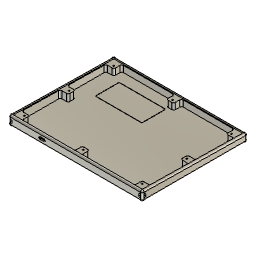
case (Autodesk Fusion 360 design; units mm, degrees)
Autodesk Fusion 360 part; units mm, degrees
sketch "Sketch1" plane through (0, 0, 0) normal (0, 0, 1) x (1, 0, 0)
  line L0 (0, 0) -> (294.692, 0)
  line L1 (294.692, 0) -> (294.692, 230.4)
  line L2 (294.692, 230.4) -> (0, 230.4)
  line L3 (0, 230.4) -> (0, 0)
  line L4 (-4, 234.4) -> (298.692, 234.4)
  line L5 (298.692, 234.4) -> (298.692, -4)
  line L6 (298.692, -4) -> (-4, -4)
  line L7 (-4, -4) -> (-4, 234.4)
  line L8 (4, 226.4) -> (290.692, 226.4)
  line L9 (290.692, 226.4) -> (290.692, 4)
  line L10 (290.692, 4) -> (4, 4)
  line L11 (4, 4) -> (4, 226.4)
  line L12 (4, 226.4) -> (20, 226.4)
  line L13 (20, 226.4) -> (20, 210.4)
  line L14 (20, 210.4) -> (4, 210.4)
  line L15 (4, 210.4) -> (4, 226.4)
  line L16 (4, 4) -> (20, 4)
  line L17 (20, 4) -> (20, 20)
  line L18 (20, 20) -> (4, 20)
  line L19 (4, 20) -> (4, 4)
  line L20 (290.692, 4) -> (274.692, 4)
  line L21 (274.692, 4) -> (274.692, 20)
  line L22 (274.692, 20) -> (290.692, 20)
  line L23 (290.692, 20) -> (290.692, 4)
  line L24 (290.692, 226.4) -> (274.692, 226.4)
  line L25 (274.692, 226.4) -> (274.692, 210.4)
  line L26 (274.692, 210.4) -> (290.692, 210.4)
  line L27 (290.692, 210.4) -> (290.692, 226.4)
  line L28 (4, 226.4) -> (290.692, 4) construction
  line L29 (4, 4) -> (290.692, 226.4) construction
  line L30 (147.346, 226.4) -> (147.346, 4) construction
  line L31 (4, 115.2) -> (290.692, 115.2) construction
  line L32 (4, 123.2) -> (20, 123.2)
  line L33 (20, 123.2) -> (20, 107.2)
  line L34 (20, 107.2) -> (4, 107.2)
  line L35 (4, 107.2) -> (4, 123.2)
  line L36 (139.346, 226.4) -> (155.346, 226.4)
  line L37 (155.346, 226.4) -> (155.346, 210.4)
  line L38 (155.346, 210.4) -> (139.346, 210.4)
  line L39 (139.346, 210.4) -> (139.346, 226.4)
  line L40 (290.692, 123.2) -> (274.692, 123.2)
  line L41 (274.692, 123.2) -> (274.692, 107.2)
  line L42 (274.692, 107.2) -> (290.692, 107.2)
  line L43 (290.692, 107.2) -> (290.692, 123.2)
  line L44 (139.346, 4) -> (155.346, 4)
  line L45 (155.346, 4) -> (155.346, 20)
  line L46 (155.346, 20) -> (139.346, 20)
  line L47 (139.346, 20) -> (139.346, 4)
  line L48 (2, 228.4) -> (292.692, 228.4)
  line L49 (292.692, 228.4) -> (292.692, 2)
  line L50 (292.692, 2) -> (2, 2)
  line L51 (2, 2) -> (2, 228.4)
  line L52 (20, 210.4) -> (2, 210.4)
  line L53 (2, 210.4) -> (2, 228.4)
  line L54 (2, 228.4) -> (20, 228.4)
  line L55 (20, 228.4) -> (20, 210.4)
  line L56 (20, 20) -> (2, 20)
  line L57 (2, 20) -> (2, 2)
  line L58 (2, 2) -> (20, 2)
  line L59 (20, 2) -> (20, 20)
  line L60 (274.692, 20) -> (292.692, 20)
  line L61 (292.692, 20) -> (292.692, 2)
  line L62 (292.692, 2) -> (274.692, 2)
  line L63 (274.692, 2) -> (274.692, 20)
  line L64 (274.692, 210.4) -> (292.692, 210.4)
  line L65 (292.692, 210.4) -> (292.692, 228.4)
  line L66 (292.692, 228.4) -> (274.692, 228.4)
  line L67 (274.692, 228.4) -> (274.692, 210.4)
  line L68 (139.346, 210.4) -> (155.346, 210.4)
  line L69 (155.346, 210.4) -> (155.346, 228.4)
  line L70 (155.346, 228.4) -> (139.346, 228.4)
  line L71 (139.346, 228.4) -> (139.346, 210.4)
  line L72 (274.692, 107.2) -> (292.692, 107.2)
  line L73 (292.692, 107.2) -> (292.692, 123.2)
  line L74 (292.692, 123.2) -> (274.692, 123.2)
  line L75 (274.692, 123.2) -> (274.692, 107.2)
  line L76 (155.346, 20) -> (139.346, 20)
  line L77 (139.346, 20) -> (139.346, 2)
  line L78 (139.346, 2) -> (155.346, 2)
  line L79 (155.346, 2) -> (155.346, 20)
  line L80 (20, 107.2) -> (2, 107.2)
  line L81 (2, 107.2) -> (2, 123.2)
  line L82 (2, 123.2) -> (20, 123.2)
  line L83 (20, 123.2) -> (20, 107.2)
  line L84 (0, 230.4) -> (37.901, 230.4) construction
  line L85 (37.901, 230.4) -> (37.901, 204.499) construction
  line L86 (37.901, 204.499) -> (0, 204.499) construction
  line L87 (0, 204.499) -> (0, 230.4) construction
  line L88 (37.901, 204.499) -> (143.109, 204.499)
  line L89 (143.109, 204.499) -> (143.109, 150.891)
  line L90 (143.109, 150.891) -> (37.901, 150.891)
  line L91 (37.901, 150.891) -> (37.901, 204.499)
  dimension "d1" = 294.692
  dimension "d2" = 230.4
  dimension "d3" = 4
  dimension "d4" = 4
  dimension "d5" = 4
  dimension "d6" = 4
  dimension "d7" = 4
  dimension "d8" = 4
  dimension "d9" = 4
  dimension "d10" = 4
  dimension "d11" = 16
  dimension "d12" = 16
  dimension "d13" = 16
  dimension "d14" = 16
  dimension "d15" = 16
  dimension "d16" = 16
  dimension "d17" = 16
  dimension "d18" = 16
  dimension "d19" = 16
  dimension "d20" = 16
  dimension "d21" = 16
  dimension "d22" = 16
  dimension "d23" = 16
  dimension "d24" = 16
  dimension "d25" = 16
  dimension "d26" = 16
  dimension "d27" = 2
  dimension "d28" = 2
  dimension "d29" = 2
  dimension "d30" = 2
  dimension "d33" = 16
  dimension "d34" = 16
  dimension "d35" = 16
  dimension "d36" = 16
  dimension "d150" = 37.901
  dimension "d151" = 25.901
  dimension "d152" = 105.208
  dimension "d153" = 53.608
  constraint horizontal L0
  constraint vertical L1
  constraint horizontal L2
  constraint vertical L3
  constraint coincident L0.start L3.end
  constraint horizontal L4
  constraint vertical L5
  constraint horizontal L6
  constraint vertical L7
  constraint horizontal L8
  constraint vertical L9
  constraint horizontal L10
  constraint vertical L11
  constraint horizontal L12
  constraint vertical L13
  constraint horizontal L14
  constraint vertical L15
  constraint horizontal L16
  constraint vertical L17
  constraint horizontal L18
  constraint vertical L19
  constraint horizontal L20
  constraint vertical L21
  constraint horizontal L22
  constraint vertical L23
  constraint horizontal L24
  constraint vertical L25
  constraint horizontal L26
  constraint vertical L27
  constraint midpoint L8 L30.start
  constraint midpoint L10 L30.end
  constraint midpoint L11 L31.start
  constraint midpoint L9 L31.end
  constraint horizontal L32
  constraint vertical L33
  constraint horizontal L34
  constraint vertical L35
  constraint coincident L11 L32.start
  constraint symmetric L31 L32 L34
  constraint horizontal L36
  constraint vertical L37
  constraint horizontal L38
  constraint vertical L39
  constraint coincident L8 L36.start
  constraint symmetric L30 L37 L39
  constraint horizontal L40
  constraint vertical L41
  constraint horizontal L42
  constraint vertical L43
  constraint coincident L9 L40.start
  constraint symmetric L31 L40 L42
  constraint horizontal L44
  constraint vertical L45
  constraint horizontal L46
  constraint vertical L47
  constraint coincident L10 L44.start
  constraint symmetric L30 L45 L47
  constraint horizontal L48
  constraint vertical L49
  constraint horizontal L50
  constraint vertical L51
  constraint horizontal L52
  constraint vertical L53
  constraint horizontal L54
  constraint vertical L55
  constraint horizontal L56
  constraint vertical L57
  constraint horizontal L58
  constraint vertical L59
  constraint horizontal L60
  constraint vertical L61
  constraint horizontal L62
  constraint vertical L63
  constraint horizontal L64
  constraint vertical L65
  constraint horizontal L66
  constraint vertical L67
  constraint horizontal L68
  constraint vertical L69
  constraint horizontal L70
  constraint vertical L71
  constraint horizontal L72
  constraint vertical L73
  constraint horizontal L74
  constraint vertical L75
  constraint coincident L49 L73.end
  constraint horizontal L76
  constraint vertical L77
  constraint horizontal L78
  constraint vertical L79
  constraint horizontal L80
  constraint vertical L81
  constraint horizontal L82
  constraint vertical L83
  constraint horizontal L84
  constraint vertical L85
  constraint horizontal L86
  constraint vertical L87
  constraint horizontal L88
  constraint vertical L89
  constraint horizontal L90
  constraint vertical L91
  measures "d1" distance of L0.start L0.end
  measures "d2" distance of L0.start L2.end
  measures "d3" distance of L3 L7
  measures "d4" distance of L2 L4
  measures "d5" distance of L0 L6
  measures "d6" distance of L1 L5
  measures "d7" distance of L3 L11
  measures "d8" distance of L2 L8
  measures "d9" distance of L1 L9
  measures "d10" distance of L0 L10
  measures "d11" distance of L8.start L12.end
  measures "d12" distance of L8.start L14.end
  measures "d13" distance of L10.end L16.end
  measures "d14" distance of L10.end L18.end
  measures "d15" distance of L9.end L20.end
  measures "d16" distance of L9.end L22.end
  measures "d17" distance of L8.end L24.end
  measures "d18" distance of L8.end L26.end
  measures "d19" distance of L32.start L32.end
  measures "d20" distance of L32.start L34.end
  measures "d21" distance of L36.start L36.end
  measures "d22" distance of L36.start L38.end
  measures "d23" distance of L40.start L40.end
  measures "d24" distance of L40.start L42.end
  measures "d25" distance of L44.start L44.end
  measures "d26" distance of L44.start L46.end
  measures "d27" distance of L3 L51
  measures "d28" distance of L2 L48
  measures "d29" distance of L0 L50
  measures "d30" distance of L1 L49
  measures "d33" distance of L38.end L37.end
  measures "d34" distance of L41.end L40.end
  measures "d35" distance of L45.end L46.end
  measures "d36" distance of L33.end L32.end
  measures "d150" distance of L2.end L84.end
  measures "d151" distance of L2.end L86.end
  measures "d152" distance of L85.end L88.end
  measures "d153" distance of L85.end L90.end
extrude "Extrude1" add sketch "Sketch1" against normal blind 1.5 contours L0 L1 L2 L3 | L4 L5 L6 L7 | L8 L11 L12 L15 L48 L51 L52 L53 L54 L55 | L8 L11 L12 L13 L14 L15 L52 L55 | L8 L48 L55 L71 | L8 L9 L10 L11 L13 L14 L17 L18 L21 L22 L25 L26 L32 L33 L34 L37 L38 L39 L40 L41 L42 L45 L46 L47 L52 L55 L56 L59 L60 L63 L64 L67 L68 L69 L71 L72 L74 L75 L76 L77 L79 L80 L82 L83 | L11 L51 L52 L82 | L8 L36 L48 L69 L70 L71 | L8 L36 L37 L38 L39 L68 L69 L71 | L11 L32 L33 L34 L35 L80 L82 L83 | L11 L35 L51 L80 L81 L82 | L8 L48 L67 L69 | L11 L51 L56 L80 | L8 L9 L24 L27 L48 L49 L64 L65 L66 L67 | L8 L9 L24 L25 L26 L27 L64 L67 | L10 L11 L16 L17 L18 L19 L56 L59 | L10 L11 L16 L19 L50 L51 L56 L57 L58 L59 | L9 L49 L64 L74 | L10 L50 L59 L77 | L9 L43 L49 L72 L73 L74 | L9 L40 L41 L42 L43 L72 L74 L75 | L10 L44 L45 L46 L47 L76 L77 L79 | L10 L44 L50 L77 L78 L79 | L9 L49 L60 L72 | L10 L50 L63 L79 | L9 L10 L20 L23 L49 L50 L60 L61 L62 L63 | L9 L10 L20 L21 L22 L23 L60 L63 | L88 L89 L90 L91 makes body 1
extrude "Extrude2" add sketch "Sketch1" along normal blind 18 contours L0 L1 L2 L3 | L4 L5 L6 L7 | L8 L11 L12 L15 L48 L51 L52 L53 L54 L55 | L8 L11 L12 L13 L14 L15 L52 L55 | L8 L36 L48 L69 L70 L71 | L8 L36 L37 L38 L39 L68 L69 L71 | L11 L32 L33 L34 L35 L80 L82 L83 | L11 L35 L51 L80 L81 L82 | L8 L9 L24 L27 L48 L49 L64 L65 L66 L67 | L8 L9 L24 L25 L26 L27 L64 L67 | L10 L11 L16 L17 L18 L19 L56 L59 | L10 L11 L16 L19 L50 L51 L56 L57 L58 L59 | L9 L43 L49 L72 L73 L74 | L9 L40 L41 L42 L43 L72 L74 L75 | L10 L44 L45 L46 L47 L76 L77 L79 | L10 L44 L50 L77 L78 L79 | L9 L10 L20 L23 L49 L50 L60 L61 L62 L63 | L9 L10 L20 L21 L22 L23 L60 L63 bodies 1
sketch "Sketch2" plane through (0, 0, 18) normal (0, 0, 1) x (-1, 0, 0)
  line L0 (-20, -123.2) -> (-2, -123.2)
  line L1 (-2, -123.2) -> (-2, -210.4)
  line L2 (-2, -210.4) -> (-20, -210.4)
  line L3 (-20, -210.4) -> (-20, -228.4)
  line L4 (-20, -228.4) -> (-139.346, -228.4)
  line L5 (-139.346, -228.4) -> (-139.346, -210.4)
  line L6 (-139.346, -210.4) -> (-155.346, -210.4)
  line L7 (-155.346, -210.4) -> (-155.346, -228.4)
  line L8 (-155.346, -228.4) -> (-274.692, -228.4)
  line L9 (-274.692, -228.4) -> (-274.692, -210.4)
  line L10 (-274.692, -210.4) -> (-292.692, -210.4)
  line L11 (-292.692, -210.4) -> (-292.692, -123.2)
  line L12 (-292.692, -123.2) -> (-274.692, -123.2)
  line L13 (-274.692, -123.2) -> (-274.692, -107.2)
  line L14 (-274.692, -107.2) -> (-292.692, -107.2)
  line L15 (-292.692, -107.2) -> (-292.692, -20)
  line L16 (-292.692, -20) -> (-274.692, -20)
  line L17 (-274.692, -20) -> (-274.692, -2)
  line L18 (-274.692, -2) -> (-155.346, -2)
  line L19 (-155.346, -2) -> (-155.346, -20)
  line L20 (-155.346, -20) -> (-139.346, -20)
  line L21 (-139.346, -20) -> (-139.346, -2)
  line L22 (-139.346, -2) -> (-20, -2)
  line L23 (-20, -2) -> (-20, -20)
  line L24 (-20, -20) -> (-2, -20)
  line L25 (-2, -20) -> (-2, -107.2)
  line L26 (-2, -107.2) -> (-20, -107.2)
  line L27 (-20, -107.2) -> (-20, -123.2)
  line L28 (4, 4) -> (-298.692, 4)
  line L29 (-298.692, 4) -> (-298.692, -234.4)
  line L30 (-298.692, -234.4) -> (4, -234.4)
  line L31 (4, -234.4) -> (4, 4)
  line L32 (-294.692, 0) -> (0, 0)
  line L33 (0, 0) -> (0, -230.4)
  line L34 (0, -230.4) -> (-294.692, -230.4)
  line L35 (-294.692, -230.4) -> (-294.692, 0)
  dimension "d39" = 4
  dimension "d40" = 4
  dimension "d41" = 4
  dimension "d42" = 4
  constraint horizontal L32
  constraint vertical L33
  constraint horizontal L34
  constraint vertical L35
  measures "d39" distance of L29 L35
  measures "d40" distance of L28 L32
  measures "d41" distance of L30 L34
  measures "d42" distance of L31 L33
sketch "Sketch3" plane through (298.692, 0, 0) normal (1, 0, 0) x (0, 1, 0)
  line L0 (-4, 18) -> (-4, -1.5)
  line L1 (-4, -1.5) -> (234.4, -1.5)
  line L2 (234.4, -1.5) -> (234.4, 18)
  line L3 (234.4, 18) -> (-4, 18)
  line L4 (234.4, -1.5) -> (234.4, 14)
  line L5 (-4, 18) -> (234.4, 14)
  dimension "d43" = 15.5
  constraint coincident L1.end L2.start
  constraint perpendicular L1 L4
  constraint coincident L0.start L3.end
  measures "d43" distance of L1.end L4.end
extrude "Extrude3" cut sketch "Sketch3" against normal through all contours L2 L3 L5 bodies 1
extrude "Extrude4" add sketch "Sketch2" along normal blind 3 separate body contours L28 L29 L30 L31 makes body 2
extrude "Extrude5" add 1 faces at (196.4613, 233.0667, 18) along direction (0, 0, -1) through all on bodies 2 bodies 1 2
sketch "Sketch4" plane through (298.692, 0, 0) normal (1, 0, 0) x (0, 1, 0)
  line L0 (234.4, -1.5) -> (234.4, 21)
  line L1 (234.4, 21) -> (-4, 21)
  line L2 (-4, 21) -> (-4, -1.5)
  line L3 (-4, -1.5) -> (234.4, -1.5)
  line L4 (234.4, -1.5) -> (234.4, 17)
  line L5 (234.4, 17) -> (-4, 21)
  dimension "d48" = 18.5
  constraint coincident L0.start L3.end
  constraint perpendicular L3 L4
  constraint coincident L1.end L2.start
  measures "d48" distance of L0.start L4.end
extrude "Extrude6" cut sketch "Sketch4" against normal through all contours L0 L1 L5 bodies 1
sketch "Sketch5" plane through (298.692, 0, 0) normal (1, 0, 0) x (0, 1, 0)
  line L0 (234.4, 17) -> (-4, 21)
  line L1 (-4, 21) -> (-4, -1.5)
  line L2 (-4, -1.5) -> (234.4, -1.5)
  line L3 (234.4, -1.5) -> (234.4, 17)
  line L4 (-4, 9.75) -> (234.4, 9.75) construction
  line L5 (-4, 13.75) -> (0, 13.75)
  line L6 (0, 13.75) -> (0, 5.75)
  line L7 (0, 5.75) -> (-4, 5.75)
  line L8 (-4, 5.75) -> (-4, 13.75)
  line L9 (-4, 13.75) -> (4, 13.75)
  line L10 (4, 13.75) -> (4, 5.75)
  line L11 (4, 5.75) -> (-4, 5.75)
  line L12 (-4, 5.75) -> (-4, 13.75)
  dimension "d50" = 4
  dimension "d51" = 8
  dimension "d52" = 8
  constraint midpoint L1 L4.start
  constraint coincident L3 L4.end
  constraint perpendicular L3 L4
  constraint horizontal L5
  constraint vertical L6
  constraint horizontal L7
  constraint vertical L8
  constraint coincident L1 L5.start
  constraint horizontal L9
  constraint vertical L10
  constraint horizontal L11
  constraint vertical L12
  constraint equal L6 L10
  constraint symmetric L4 L5 L7
  measures "d50" distance of L5.start L5.end
  measures "d51" distance of L5.start L7.end
  measures "d52" distance of L5.start L9.end
sketch "Sketch6" plane through (0, -4, 0) normal (0, -1, 0) x (1, 0, 0)
  line L0 (-4, 21) -> (-4, -1.5)
  line L1 (-4, -1.5) -> (298.692, -1.5)
  line L2 (298.692, -1.5) -> (298.692, 21)
  line L3 (298.692, 21) -> (-4, 21)
  line L4 (298.692, 21) -> (-4, -1.5) construction
  line L5 (-4, 21) -> (298.692, -1.5) construction
  line L6 (147.346, -1.5) -> (147.346, 21) construction
  line L7 (147.346, 21) -> (-4, -1.5) construction
  line L8 (-4, 21) -> (147.346, -1.5) construction
  line L9 (-4, 9.75) -> (147.346, 9.75) construction
  line L10 (-4, 13.75) -> (0, 13.75)
  line L11 (0, 13.75) -> (0, 5.75)
  line L12 (0, 5.75) -> (-4, 5.75)
  line L13 (-4, 5.75) -> (-4, 13.75)
  line L14 (-4, 13.75) -> (4, 13.75)
  line L15 (4, 13.75) -> (4, 5.75)
  line L16 (4, 5.75) -> (-4, 5.75)
  line L17 (-4, 5.75) -> (-4, 13.75)
  line L18 (298.692, 9.75) -> (147.346, 9.75) construction
  line L19 (298.692, 13.75) -> (294.692, 13.75)
  line L20 (294.692, 13.75) -> (294.692, 5.75)
  line L21 (294.692, 5.75) -> (298.692, 5.75)
  line L22 (298.692, 5.75) -> (298.692, 13.75)
  line L23 (298.692, 13.75) -> (290.692, 13.75)
  line L24 (290.692, 13.75) -> (290.692, 5.75)
  line L25 (290.692, 5.75) -> (298.692, 5.75)
  line L26 (298.692, 5.75) -> (298.692, 13.75)
  line L27 (62.173, 12.5) -> (81.173, 12.5)
  line L28 (81.173, 12.5) -> (81.173, 7)
  line L29 (81.173, 7) -> (62.173, 7)
  line L30 (62.173, 7) -> (62.173, 12.5)
  line L31 (71.673, 9.75) -> (71.673, -1.5) construction
  line L32 (66.173, 12.5) -> (77.173, 12.5)
  line L33 (77.173, 12.5) -> (77.173, 7)
  line L34 (77.173, 7) -> (66.173, 7)
  line L35 (66.173, 7) -> (66.173, 12.5)
  circle A0 centre (64.423, 9.7337) radius 1
  circle A1 centre (78.923, 9.7337) radius 1
  dimension "d53" = 4
  dimension "d54" = 8
  dimension "d55" = 8
  dimension "d67" = 4
  dimension "d68" = 8
  dimension "d69" = 8
  dimension "d158" = 19
  dimension "d159" = 5.5
  dimension "d160" = 11
  dimension "d161" = 2
  dimension "d162" = 2
  dimension "d177" = 14.5
  constraint coincident L2.end L3.start
  constraint coincident L0.end L1.start
  constraint coincident L0.start L3.end
  constraint coincident L1.end L2.start
  constraint midpoint L1 L6.start
  constraint midpoint L3 L6.end
  constraint midpoint L0 L9.start
  constraint midpoint L6 L9.end
  constraint horizontal L10
  constraint vertical L11
  constraint horizontal L12
  constraint vertical L13
  constraint coincident L0 L10.start
  constraint horizontal L14
  constraint vertical L15
  constraint horizontal L16
  constraint vertical L17
  constraint equal L11 L15
  constraint symmetric L9 L10 L12
  constraint midpoint L2 L18.start
  constraint horizontal L19
  constraint vertical L20
  constraint horizontal L21
  constraint vertical L22
  constraint coincident L2 L19.start
  constraint horizontal L23
  constraint vertical L24
  constraint horizontal L25
  constraint vertical L26
  constraint equal L20 L24
  constraint symmetric L18 L19 L21
  constraint horizontal L27
  constraint vertical L28
  constraint horizontal L29
  constraint vertical L30
  constraint midpoint L9 L31.start
  constraint coincident L1 L31.end
  constraint perpendicular L1 L31
  constraint symmetric L28 L30 L31
  constraint symmetric L9 L27 L29
  constraint horizontal L32
  constraint vertical L33
  constraint horizontal L34
  constraint vertical L35
  constraint coincident L27 L32.start
  constraint equal L30 L35
  constraint symmetric L31 L33 L35
  constraint symmetric L31 A0.centre A1.centre
  measures "d53" distance of L10.start L10.end
  measures "d54" distance of L10.start L12.end
  measures "d55" distance of L10.start L14.end
  measures "d67" distance of L19.start L19.end
  measures "d68" distance of L19.start L21.end
  measures "d69" distance of L19.start L23.end
  measures "d158" distance of L27.start L27.end
  measures "d159" distance of L27.start L29.end
  measures "d160" distance of L32.start L32.end
  measures "d161" diameter of A0
  measures "d162" diameter of A1
  measures "d177" distance of A0.centre A1.centre
sketch "Sketch7" plane through (-4, 0, 0) normal (-1, 0, 0) x (0, -1, 0)
  line L0 (4, 21) -> (-234.4, 17)
  line L1 (-234.4, 17) -> (-234.4, -1.5)
  line L2 (-234.4, -1.5) -> (4, -1.5)
  line L3 (4, -1.5) -> (4, 21)
  line L4 (4, 9.75) -> (-234.4, 9.75) construction
  line L5 (4, 13.75) -> (0, 13.75)
  line L6 (0, 13.75) -> (0, 5.75)
  line L7 (0, 5.75) -> (4, 5.75)
  line L8 (4, 5.75) -> (4, 13.75)
  line L9 (4, 13.75) -> (-4, 13.75)
  line L10 (-4, 13.75) -> (-4, 5.75)
  line L11 (-4, 5.75) -> (4, 5.75)
  line L12 (4, 5.75) -> (4, 13.75)
  dimension "d58" = 4
  dimension "d59" = 8
  dimension "d60" = 8
  constraint midpoint L3 L4.start
  constraint coincident L1 L4.end
  constraint perpendicular L1 L4
  constraint horizontal L5
  constraint vertical L6
  constraint horizontal L7
  constraint vertical L8
  constraint coincident L3 L5.start
  constraint horizontal L9
  constraint vertical L10
  constraint horizontal L11
  constraint vertical L12
  constraint equal L6 L10
  constraint symmetric L4 L5 L7
  measures "d58" distance of L5.start L5.end
  measures "d59" distance of L5.start L7.end
  measures "d60" distance of L5.start L9.end
fillet "Fillet1" radius 4 28 edges at (20, 228.4, 7.0503) (20, 210.4, 7.2013) (2, 210.4, 7.2013) (20, 123.2, 7.9329) (2, 123.2, 7.9329) (2, 107.2, 8.0671) (20, 107.2, 8.0671) (2, 20, 8.7987) (20, 20, 8.7987) (20, 2, 8.9497) (139.346, 20, 8.7987) (139.346, 2, 8.9497) (155.346, 20, 8.7987) (155.346, 2, 8.9497) (274.692, 20, 8.7987) (274.692, 2, 8.9497) (292.692, 20, 8.7987) (292.692, 107.2, 8.0671) (274.692, 107.2, 8.0671) (274.692, 123.2, 7.9329) (292.692, 123.2, 7.9329) (292.692, 210.4, 7.2013) (274.692, 210.4, 7.2013) (274.692, 228.4, 7.0503) (155.346, 228.4, 7.0503) (139.346, 228.4, 7.0503) (139.346, 210.4, 7.2013) (155.346, 210.4, 7.2013) on bodies 1
fillet "Fillet2" radius 2 4 edges at (294.692, 230.4, 15.5671) (0, 230.4, 15.5671) (0, 0, 19.4329) (294.692, 0, 19.4329) on bodies 1
fillet "Fillet3" radius 4 4 edges at (-4, -4, 9.75) (298.692, -4, 9.75) (-4, 234.4, 7.75) (298.692, 234.4, 7.75) on bodies 1
extrude "Extrude8" cut sketch "Sketch7" against normal blind 4 contours L6 L9 L10 L11 bodies 1
extrude "Extrude9" cut sketch "Sketch6" against normal blind 8 contours L11 L14 L15 L16 bodies 1
extrude "Extrude10" cut sketch "Sketch5" against normal blind 4 contours L6 L9 L10 L11 bodies 1
extrude "Extrude11" cut sketch "Sketch6" against normal blind 8 contours L20 L23 L24 L25 bodies 1
fillet "Fillet4" radius 2 5 edges at (290.692, 0, 13.75) (294.692, 4, 13.75) (290.692, 0, 5.75) (294.692, 4, 5.75) (290.692, 4, 9.75) on bodies 1
fillet "Fillet5" radius 2 5 edges at (0, 4, 13.75) (4, 0, 13.75) (0, 4, 5.75) (4, 0, 5.75) (4, 4, 9.75) on bodies 1
fillet "Fillet6" radius 4 16 edges at (297.5204, -2.8284, 20.9803) (298.692, 115.2, 19) (297.5204, 233.2284, 17.0197) (147.346, 234.4, 17) (-2.8284, 233.2284, 17.0197) (-4, 115.2, 19) (-2.8284, -2.8284, 20.9803) (147.346, -4, 21) (-2.8284, -2.8284, -1.5) (-4, 115.2, -1.5) (-2.8284, 233.2284, -1.5) (147.346, 234.4, -1.5) (297.5204, 233.2284, -1.5) (298.692, 115.2, -1.5) (297.5204, -2.8284, -1.5) (147.346, -4, -1.5) on bodies 1
hole "Hole1" at (280.692, 14.0008, 17.698) direction (0, -0.016776, -0.999859) diameter 3.332 depth 10 tip angle 118 bodies 1
thread "Thread1" "ISO Metric profile 4.0 M4x0.7 6H" thread offset 0 thread depth 7.4
hole "Hole2" at (147.346, 14.0008, 17.698) direction (0, -0.016776, -0.999859) diameter 3.332 depth 10 tip angle 118 bodies 1
thread "Thread2" "ISO Metric profile 4.0 M4x0.7 6H" thread offset 0 thread depth 7.4
hole "Hole3" at (14, 14.0008, 17.698) direction (0, -0.016776, -0.999859) diameter 3.332 depth 10 tip angle 118 bodies 1
thread "Thread3" "ISO Metric profile 4.0 M4x0.7 6H" thread offset 0 thread depth 7.4
hole "Hole4" at (280.692, 115.1989, 16) direction (0, -0.016776, -0.999859) diameter 3.332 depth 10 tip angle 118 bodies 1
thread "Thread4" "ISO Metric profile 4.0 M4x0.7 6H" thread offset 0 thread depth 7.4
hole "Hole5" at (14, 115.1989, 16) direction (0, -0.016776, -0.999859) diameter 3.332 depth 10 tip angle 118 bodies 1
thread "Thread5" "ISO Metric profile 4.0 M4x0.7 6H" thread offset 0 thread depth 7.4
hole "Hole6" at (280.692, 216.3992, 14.302) direction (0, -0.016776, -0.999859) diameter 3.332 depth 10 tip angle 118 bodies 1
thread "Thread6" "ISO Metric profile 4.0 M4x0.7 6H" thread offset 0 thread depth 7.4
hole "Hole7" at (147.346, 216.3992, 14.302) direction (0, -0.016776, -0.999859) diameter 3.332 depth 10 tip angle 118 bodies 1
thread "Thread7" "ISO Metric profile 4.0 M4x0.7 6H" thread offset 0 thread depth 7.4
hole "Hole8" at (14, 216.3992, 14.302) direction (0, -0.016776, -0.999859) diameter 3.332 depth 10 tip angle 118 bodies 1
thread "Thread8" "ISO Metric profile 4.0 M4x0.7 6H" thread offset 0 thread depth 7.4
extrude "Extrude13" cut sketch "Sketch1" against normal blind 0.5 contours L88 L89 L90 L91 bodies 1
fillet "Fillet8" radius 2 4 edges at (37.901, 204.499, -0.25) (37.901, 150.891, -0.25) (143.109, 150.891, -0.25) (143.109, 204.499, -0.25) on bodies 1
extrude "Extrude14" cut sketch "Sketch6" against normal blind 6 contours L27 L29 L32 L33 L34 L35 bodies 1
extrude "Extrude15" cut sketch "Sketch6" against normal blind 6 contours A0 | A1 bodies 1
fillet "Fillet9" radius 1.05 4 edges at (66.173, -1, 12.5) (66.173, -1, 7) (77.173, -1, 12.5) (77.173, -1, 7) on bodies 1
sketch "Sketch8" plane through (0, 2, 0) normal (0, 1, 0) x (-1, 0, 0)
  circle A0 centre (-64.423, 9.7337) radius 1
  circle A1 centre (-78.923, 9.7337) radius 1
  line L0 (-77.173, 8.05) -> (-77.173, 11.45)
  arc A2 (-76.123, 12.5) -> (-77.173, 11.45) centre (-76.123, 11.45) ccw
  line L1 (-76.123, 12.5) -> (-67.223, 12.5)
  arc A3 (-66.173, 11.45) -> (-67.223, 12.5) centre (-67.223, 11.45) ccw
  line L2 (-66.173, 11.45) -> (-66.173, 8.05)
  arc A4 (-67.223, 7) -> (-66.173, 8.05) centre (-67.223, 8.05) ccw
  line L3 (-67.223, 7) -> (-76.123, 7)
  arc A5 (-77.173, 8.05) -> (-76.123, 7) centre (-76.123, 8.05) ccw
  line L4 (-135.346, 17.8993) -> (-135.346, 0)
  line L5 (-135.346, 0) -> (-24, 0)
  line L6 (-24, 0) -> (-24, 17.8993)
  line L7 (-24, 17.8993) -> (-135.346, 17.8993)
  line L8 (-83.173, 14.5) -> (-60.173, 14.5)
  line L9 (-60.173, 14.5) -> (-60.173, 5)
  line L10 (-60.173, 5) -> (-83.173, 5)
  line L11 (-83.173, 5) -> (-83.173, 14.5)
  dimension "d169" = 2
  dimension "d170" = 2
  dimension "d171" = 4.25
  dimension "d172" = 4.25
  constraint horizontal L8
  constraint vertical L9
  constraint horizontal L10
  constraint vertical L11
  measures "d169" distance of L1 L8
  measures "d170" distance of L3 L10
  measures "d171" distance of A1.centre L11
  measures "d172" distance of A0.centre L9
extrude "Extrude16" cut sketch "Sketch8" against normal blind 3 contours L8 L9 L10 L11 bodies 1
fillet "Fillet10" radius 2 4 edges at (83.173, 0.5, 14.5) (60.173, 0.5, 14.5) (60.173, 0.5, 5) (83.173, 0.5, 5) on bodies 1
fillet "Fillet11" radius 2 4 edges at (0, -2, 13.75) (-2, 0, 13.75) (-2, 0, 5.75) (0, -2, 5.75) on bodies 1
fillet "Fillet12" radius 2 4 edges at (294.692, -2, 5.75) (294.692, -2, 13.75) (296.692, 0, 13.75) (296.692, 0, 5.75) on bodies 1
equation "d43 = 14 mm + 1.5 mm"
equation "d48 = 14 mm + 3 mm + 1.5 mm"
equation "d150 = 37.701 mm + 0.2 mm"
equation "d151 = 25.701 mm + 0.2 mm"
